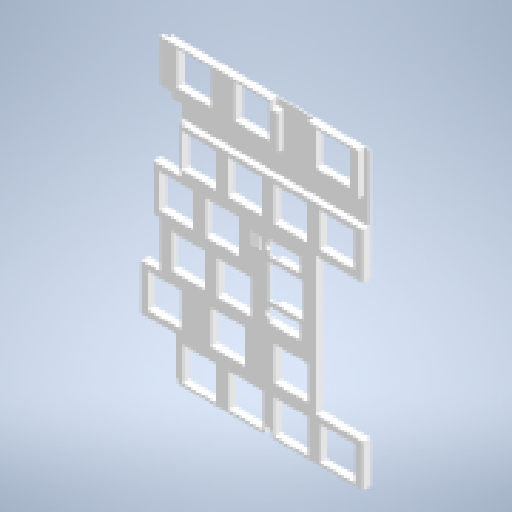
# Autodesk Inventor part: Right Plate
Saved by Autodesk Inventor 2025 (Build 290162000, 162)
## iProperties
Created: 2024-08-15
Part Number: Right Plate
Material: PBT Plastic
Document SubType Name: Modeling
Designer: adam
Density: 1.31 g/cm^3
Appearance: Smooth - White
Author: adam
Autodesk Inventor part; units mm, degrees
ref_plane "YZ Plane" through (0, 0, 0) normal (1, 0, 0) x (0, 1, 0)
ref_plane "XZ Plane" through (0, 0, 0) normal (0, 1, 0) x (-1, 0, 0)
ref_plane "XY Plane" through (0, 0, 0) normal (0, 0, 1) x (1, 0, 0)
sketch "Sketch1" plane through (0, 0, 0) normal (0, 0, 1) x (1, 0, 0)
  line L0 (356, -163) -> (40, -163) construction
  line L1 (356, -42) -> (356, -163) construction
  line L2 (40, -42) -> (356, -42) projected
  line L3 (40, -163) -> (40, -42) construction
  circle A0 centre (58.6, -159.6) radius 0.725 construction
  circle A1 centre (63, -154.9) radius 2.55 construction
  circle A2 centre (65.6, -160.65) radius 0.725 construction
  circle A3 centre (83.1, -159.6) radius 0.725 construction
  circle A4 centre (90.1, -160.65) radius 0.725 construction
  circle A5 centre (87.5, -154.9) radius 2.55 construction
  line L4 (107.125, -161.9) -> (113.125, -161.9) construction
  line L5 (107.125, -145.9) -> (107.125, -161.9) construction
  line L6 (113.125, -145.9) -> (107.125, -145.9) construction
  line L7 (113.125, -161.9) -> (113.125, -145.9) construction
  circle A6 centre (53.1, -140.5) radius 0.725 construction
  circle A7 centre (60.1, -141.55) radius 0.725 construction
  circle A8 centre (79.35, -140.5) radius 0.725 construction
  circle A9 centre (57.5, -135.8) radius 2.55 construction
  circle A10 centre (86.35, -141.55) radius 0.725 construction
  circle A11 centre (98.35, -140.5) radius 0.725 construction
  circle A12 centre (105.35, -141.55) radius 0.725 construction
  circle A13 centre (117.35, -140.5) radius 0.725 construction
  circle A14 centre (83.75, -135.8) radius 2.55 construction
  circle A15 centre (102.75, -135.8) radius 2.55 construction
  circle A16 centre (121.75, -135.8) radius 2.55 construction
  circle A17 centre (179.475, -160.65) radius 0.725 construction
  circle A18 centre (172.475, -159.6) radius 0.725 construction
  circle A19 centre (176.875, -154.9) radius 2.55 construction
  circle A20 centre (124.35, -141.55) radius 0.725 construction
  circle A21 centre (136.35, -140.5) radius 0.725 construction
  circle A22 centre (143.35, -141.55) radius 0.725 construction
  circle A23 centre (155.35, -140.5) radius 0.725 construction
  circle A24 centre (140.75, -135.8) radius 2.55 construction
  circle A25 centre (159.75, -135.8) radius 2.55 construction
  circle A26 centre (162.35, -141.55) radius 0.725 construction
  circle A27 centre (174.35, -140.5) radius 0.725 construction
  circle A28 centre (181.35, -141.55) radius 0.725 construction
  circle A29 centre (193.35, -140.5) radius 0.725 construction
  circle A30 centre (178.75, -135.8) radius 2.55 construction
  circle A31 centre (197.75, -135.8) radius 2.55 construction
  circle A32 centre (48.6, -121.4) radius 0.725 construction
  circle A33 centre (55.6, -122.45) radius 0.725 construction
  circle A34 centre (70.1, -121.4) radius 0.725 construction
  circle A35 centre (77.1, -122.45) radius 0.725 construction
  circle A36 centre (89.1, -121.4) radius 0.725 construction
  circle A37 centre (96.1, -122.45) radius 0.725 construction
  circle A38 centre (108.1, -121.4) radius 0.725 construction
  circle A39 centre (115.1, -122.45) radius 0.725 construction
  circle A40 centre (53, -116.7) radius 2.55 construction
  circle A41 centre (74.5, -116.7) radius 2.55 construction
  circle A42 centre (93.5, -116.7) radius 2.55 construction
  circle A43 centre (112.5, -116.7) radius 2.55 construction
  circle A44 centre (127.1, -121.4) radius 0.725 construction
  circle A45 centre (134.1, -122.45) radius 0.725 construction
  circle A46 centre (146.1, -121.4) radius 0.725 construction
  circle A47 centre (153.1, -122.45) radius 0.725 construction
  circle A48 centre (165.1, -121.4) radius 0.725 construction
  circle A49 centre (172.1, -122.45) radius 0.725 construction
  circle A50 centre (184.1, -121.4) radius 0.725 construction
  circle A51 centre (191.1, -122.45) radius 0.725 construction
  circle A52 centre (131.5, -116.7) radius 2.55 construction
  circle A53 centre (150.5, -116.7) radius 2.55 construction
  circle A54 centre (169.5, -116.7) radius 2.55 construction
  circle A55 centre (188.5, -116.7) radius 2.55 construction
  circle A56 centre (261.85, -159.6) radius 0.725 construction
  circle A57 centre (268.85, -160.65) radius 0.725 construction
  circle A58 centre (266.25, -154.9) radius 2.55 construction
  line L8 (240.625, -161.9) -> (246.625, -161.9) construction
  line L9 (240.625, -145.9) -> (240.625, -161.9) construction
  line L10 (246.625, -145.9) -> (240.625, -145.9) construction
  line L11 (246.625, -161.9) -> (246.625, -145.9) construction
  circle A59 centre (200.35, -141.55) radius 0.725 construction
  circle A60 centre (212.35, -140.5) radius 0.725 construction
  circle A61 centre (219.35, -141.55) radius 0.725 construction
  circle A62 centre (231.35, -140.5) radius 0.725 construction
  circle A63 centre (216.75, -135.8) radius 2.55 construction
  circle A64 centre (235.75, -135.8) radius 2.55 construction
  circle A65 centre (238.35, -141.55) radius 0.725 construction
  circle A66 centre (250.35, -140.5) radius 0.725 construction
  circle A67 centre (257.35, -141.55) radius 0.725 construction
  circle A68 centre (269.35, -140.5) radius 0.725 construction
  circle A69 centre (276.35, -141.55) radius 0.725 construction
  circle A70 centre (254.75, -135.8) radius 2.55 construction
  circle A71 centre (273.75, -135.8) radius 2.55 construction
  circle A72 centre (283.85, -159.6) radius 0.725 construction
  circle A73 centre (290.85, -160.65) radius 0.725 construction
  circle A74 centre (288.25, -154.9) radius 2.55 construction
  circle A75 centre (302.85, -159.6) radius 0.725 construction
  circle A76 centre (309.85, -160.65) radius 0.725 construction
  circle A77 centre (307.25, -154.9) radius 2.55 construction
  circle A78 centre (321.85, -159.6) radius 0.725 construction
  circle A79 centre (328.85, -160.65) radius 0.725 construction
  circle A80 centre (326.25, -154.9) radius 2.55 construction
  circle A81 centre (340.85, -159.6) radius 0.725 construction
  circle A82 centre (347.85, -160.65) radius 0.725 construction
  circle A83 centre (345.25, -154.9) radius 2.55 construction
  circle A84 centre (295.6, -140.5) radius 0.725 construction
  circle A85 centre (302.6, -141.55) radius 0.725 construction
  circle A86 centre (300, -135.8) radius 2.55 construction
  circle A87 centre (321.85, -140.5) radius 0.725 construction
  circle A88 centre (328.85, -141.55) radius 0.725 construction
  circle A89 centre (353.5, -141.62) radius 0.5 construction
  circle A90 centre (326.25, -135.8) radius 2.55 construction
  circle A91 centre (353.5, -139.08) radius 0.5 construction
  circle A92 centre (353.5, -136.54) radius 0.5 construction
  circle A93 centre (353.5, -134) radius 0.5 construction
  circle A94 centre (203.1, -121.4) radius 0.725 construction
  circle A95 centre (210.1, -122.45) radius 0.725 construction
  circle A96 centre (222.1, -121.4) radius 0.725 construction
  circle A97 centre (229.1, -122.45) radius 0.725 construction
  circle A98 centre (241.1, -121.4) radius 0.725 construction
  circle A99 centre (248.1, -122.45) radius 0.725 construction
  circle A100 centre (260.1, -121.4) radius 0.725 construction
  circle A101 centre (267.1, -122.45) radius 0.725 construction
  circle A102 centre (207.5, -116.7) radius 2.55 construction
  circle A103 centre (226.5, -116.7) radius 2.55 construction
  circle A104 centre (245.5, -116.7) radius 2.55 construction
  circle A105 centre (264.5, -116.7) radius 2.55 construction
  circle A106 centre (279.1, -121.4) radius 0.725 construction
  circle A107 centre (286.1, -122.45) radius 0.725 construction
  circle A108 centre (298.1, -121.4) radius 0.725 construction
  circle A109 centre (305.1, -122.45) radius 0.725 construction
  line L12 (315, -122.25) -> (330, -122.25) construction
  line L13 (315, -116.25) -> (315, -122.25) construction
  line L14 (330, -116.25) -> (315, -116.25) construction
  line L15 (330, -122.25) -> (330, -116.25) construction
  circle A110 centre (283.5, -116.7) radius 2.55 construction
  circle A111 centre (302.5, -116.7) radius 2.55 construction
  circle A112 centre (328.675, -111.675) radius 0.725 construction
  circle A113 centre (323.975, -107.275) radius 2.55 construction
  circle A114 centre (329.725, -104.675) radius 0.725 construction
  circle A115 centre (62.6, -103.35) radius 0.725 construction
  circle A116 centre (55.6, -102.3) radius 0.725 construction
  circle A117 centre (60, -97.6) radius 2.55 construction
  line L16 (45, -103.6) -> (51, -103.6) construction
  line L17 (45, -88.6) -> (45, -103.6) construction
  line L18 (51, -88.6) -> (45, -88.6) construction
  line L19 (51, -103.6) -> (51, -88.6) construction
  line L20 (69, -103.6) -> (75, -103.6) construction
  line L21 (69, -88.6) -> (69, -103.6) construction
  line L22 (75, -88.6) -> (69, -88.6) construction
  line L23 (75, -103.6) -> (75, -88.6) construction
  circle A118 centre (91.35, -103.35) radius 0.725 construction
  circle A119 centre (84.35, -102.3) radius 0.725 construction
  circle A120 centre (88.75, -97.6) radius 2.55 construction
  circle A121 centre (110.35, -103.35) radius 0.725 construction
  circle A122 centre (103.35, -102.3) radius 0.725 construction
  circle A123 centre (107.75, -97.6) radius 2.55 construction
  circle A124 centre (57.6, -84.25) radius 0.725 construction
  circle A125 centre (81.6, -84.25) radius 0.725 construction
  circle A126 centre (50.6, -83.2) radius 0.725 construction
  circle A127 centre (55, -78.5) radius 2.55 construction
  circle A128 centre (74.6, -83.2) radius 0.725 construction
  circle A129 centre (79, -78.5) radius 2.55 construction
  circle A130 centre (100.6, -84.25) radius 0.725 construction
  circle A131 centre (119.6, -84.25) radius 0.725 construction
  circle A132 centre (93.6, -83.2) radius 0.725 construction
  circle A133 centre (98, -78.5) radius 2.55 construction
  circle A134 centre (112.6, -83.2) radius 0.725 construction
  circle A135 centre (117, -78.5) radius 2.55 construction
  circle A136 centre (129.35, -103.35) radius 0.725 construction
  circle A137 centre (122.35, -102.3) radius 0.725 construction
  circle A138 centre (141.35, -102.3) radius 0.725 construction
  circle A139 centre (126.75, -97.6) radius 2.55 construction
  circle A140 centre (148.35, -103.35) radius 0.725 construction
  circle A141 centre (160.35, -102.3) radius 0.725 construction
  circle A142 centre (145.75, -97.6) radius 2.55 construction
  circle A143 centre (167.35, -103.35) radius 0.725 construction
  circle A144 centre (179.35, -102.3) radius 0.725 construction
  circle A145 centre (164.75, -97.6) radius 2.55 construction
  circle A146 centre (186.35, -103.35) radius 0.725 construction
  circle A147 centre (198.35, -102.3) radius 0.725 construction
  circle A148 centre (183.75, -97.6) radius 2.55 construction
  circle A149 centre (138.6, -84.25) radius 0.725 construction
  circle A150 centre (157.6, -84.25) radius 0.725 construction
  circle A151 centre (131.6, -83.2) radius 0.725 construction
  circle A152 centre (136, -78.5) radius 2.55 construction
  circle A153 centre (150.6, -83.2) radius 0.725 construction
  circle A154 centre (155, -78.5) radius 2.55 construction
  circle A155 centre (176.6, -84.25) radius 0.725 construction
  circle A156 centre (195.6, -84.25) radius 0.725 construction
  circle A157 centre (169.6, -83.2) radius 0.725 construction
  circle A158 centre (174, -78.5) radius 2.55 construction
  circle A159 centre (188.6, -83.2) radius 0.725 construction
  circle A160 centre (193, -78.5) radius 2.55 construction
  circle A161 centre (48.1, -54.7) radius 0.725 construction
  circle A162 centre (55.1, -55.75) radius 0.725 construction
  circle A163 centre (81.1, -54.7) radius 0.725 construction
  circle A164 centre (52.5, -50) radius 2.55 construction
  circle A165 centre (88.1, -55.75) radius 0.725 construction
  circle A166 centre (105.1, -54.7) radius 0.725 construction
  circle A167 centre (112.1, -55.75) radius 0.725 construction
  circle A168 centre (85.5, -50) radius 2.55 construction
  circle A169 centre (109.5, -50) radius 2.55 construction
  circle A170 centre (163.5, -66.25) radius 0.425 construction
  circle A171 centre (166, -66.25) radius 0.425 construction
  circle A172 centre (168.5, -66.25) radius 0.425 construction
  circle A173 centre (171, -66.25) radius 0.425 construction
  circle A174 centre (173.5, -66.25) radius 0.425 construction
  circle A175 centre (176, -66.25) radius 0.425 construction
  circle A176 centre (178.5, -66.25) radius 0.425 construction
  circle A177 centre (162.25, -63.75) radius 0.425 construction
  circle A178 centre (164.75, -63.75) radius 0.425 construction
  circle A179 centre (167.25, -63.75) radius 0.425 construction
  circle A180 centre (169.75, -63.75) radius 0.425 construction
  circle A181 centre (172.25, -63.75) radius 0.425 construction
  circle A182 centre (174.75, -63.75) radius 0.425 construction
  circle A183 centre (177.25, -63.75) radius 0.425 construction
  circle A184 centre (179.75, -63.75) radius 0.425 construction
  circle A185 centre (181, -66.25) radius 0.425 construction
  circle A186 centre (183.5, -66.25) radius 0.425 construction
  circle A187 centre (186, -66.25) radius 0.425 construction
  circle A188 centre (188.5, -66.25) radius 0.425 construction
  circle A189 centre (191, -66.25) radius 0.425 construction
  circle A190 centre (193.5, -66.25) radius 0.425 construction
  circle A191 centre (196, -66.25) radius 0.425 construction
  circle A192 centre (198.5, -66.25) radius 0.425 construction
  circle A193 centre (182.25, -63.75) radius 0.425 construction
  circle A194 centre (184.75, -63.75) radius 0.425 construction
  circle A195 centre (187.25, -63.75) radius 0.425 construction
  circle A196 centre (189.75, -63.75) radius 0.425 construction
  circle A197 centre (192.25, -63.75) radius 0.425 construction
  circle A198 centre (194.75, -63.75) radius 0.425 construction
  circle A199 centre (197.25, -63.75) radius 0.425 construction
  circle A200 centre (129.1, -54.7) radius 0.725 construction
  circle A201 centre (136.1, -55.75) radius 0.725 construction
  circle A202 centre (153.1, -54.7) radius 0.725 construction
  circle A203 centre (160.1, -55.75) radius 0.725 construction
  circle A204 centre (133.5, -50) radius 2.55 construction
  circle A205 centre (157.5, -50) radius 2.55 construction
  circle A206 centre (177.1, -54.7) radius 0.725 construction
  circle A207 centre (184.1, -55.75) radius 0.725 construction
  circle A208 centre (181.5, -50) radius 2.55 construction
  circle A209 centre (205.35, -103.35) radius 0.725 construction
  circle A210 centre (217.35, -102.3) radius 0.725 construction
  circle A211 centre (202.75, -97.6) radius 2.55 construction
  circle A212 centre (224.35, -103.35) radius 0.725 construction
  circle A213 centre (236.35, -102.3) radius 0.725 construction
  circle A214 centre (221.75, -97.6) radius 2.55 construction
  circle A215 centre (243.35, -103.35) radius 0.725 construction
  circle A216 centre (255.35, -102.3) radius 0.725 construction
  circle A217 centre (240.75, -97.6) radius 2.55 construction
  circle A218 centre (262.35, -103.35) radius 0.725 construction
  circle A219 centre (274.35, -102.3) radius 0.725 construction
  circle A220 centre (259.75, -97.6) radius 2.55 construction
  circle A221 centre (214.6, -84.25) radius 0.725 construction
  circle A222 centre (233.6, -84.25) radius 0.725 construction
  circle A223 centre (207.6, -83.2) radius 0.725 construction
  circle A224 centre (212, -78.5) radius 2.55 construction
  circle A225 centre (226.6, -83.2) radius 0.725 construction
  circle A226 centre (231, -78.5) radius 2.55 construction
  circle A227 centre (252.6, -84.25) radius 0.725 construction
  circle A228 centre (271.6, -84.25) radius 0.725 construction
  circle A229 centre (245.6, -83.2) radius 0.725 construction
  circle A230 centre (250, -78.5) radius 2.55 construction
  circle A231 centre (264.6, -83.2) radius 0.725 construction
  circle A232 centre (269, -78.5) radius 2.55 construction
  circle A233 centre (281.35, -103.35) radius 0.725 construction
  circle A234 centre (293.35, -102.3) radius 0.725 construction
  circle A235 centre (278.75, -97.6) radius 2.55 construction
  circle A236 centre (300.35, -103.35) radius 0.725 construction
  circle A237 centre (297.75, -97.6) radius 2.55 construction
  line L24 (315, -98.25) -> (330, -98.25) construction
  line L25 (315, -92.25) -> (315, -98.25) construction
  line L26 (330, -92.25) -> (315, -92.25) construction
  line L27 (330, -98.25) -> (330, -92.25) construction
  circle A238 centre (290.6, -84.25) radius 0.725 construction
  circle A239 centre (309.6, -84.25) radius 0.725 construction
  circle A240 centre (283.6, -83.2) radius 0.725 construction
  circle A241 centre (288, -78.5) radius 2.55 construction
  circle A242 centre (302.6, -83.2) radius 0.725 construction
  circle A243 centre (307, -78.5) radius 2.55 construction
  circle A244 centre (328.6, -84.25) radius 0.725 construction
  circle A245 centre (347.6, -84.25) radius 0.725 construction
  circle A246 centre (321.6, -83.2) radius 0.725 construction
  circle A247 centre (326, -78.5) radius 2.55 construction
  circle A248 centre (340.6, -83.2) radius 0.725 construction
  circle A249 centre (345, -78.5) radius 2.55 construction
  circle A250 centre (201, -66.25) radius 0.425 construction
  circle A251 centre (199.75, -63.75) radius 0.425 construction
  circle A252 centre (259, -74) radius 1.6 construction
  circle A253 centre (209.6, -54.7) radius 0.725 construction
  circle A254 centre (216.6, -55.75) radius 0.725 construction
  circle A255 centre (233.6, -54.7) radius 0.725 construction
  circle A256 centre (214, -50) radius 2.55 construction
  circle A257 centre (238, -50) radius 2.55 construction
  circle A258 centre (240.6, -55.75) radius 0.725 construction
  circle A259 centre (257.6, -54.7) radius 0.725 construction
  circle A260 centre (264.6, -55.75) radius 0.725 construction
  circle A261 centre (262, -50) radius 2.55 construction
  circle A262 centre (281.6, -54.7) radius 0.725 construction
  circle A263 centre (288.6, -55.75) radius 0.725 construction
  circle A264 centre (305.6, -54.7) radius 0.725 construction
  circle A265 centre (312.6, -55.75) radius 0.725 construction
  circle A266 centre (286, -50) radius 2.55 construction
  circle A267 centre (310, -50) radius 2.55 construction
  circle A268 centre (339.1, -54.7) radius 0.725 construction
  circle A269 centre (346.1, -55.75) radius 0.725 construction
  circle A270 centre (343.5, -50) radius 2.55 construction
  line L28 (274, -42) -> (274, -64.25) projected
  line L29 (274, -64.25) -> (278.5, -64.25) projected
  line L30 (278.5, -88.05) -> (278.5, -64.25) projected
  line L31 (269.25, -88.05) -> (278.5, -88.05) projected
  line L32 (269.25, -107.15) -> (269.25, -88.05) projected
  line L33 (274, -107.15) -> (269.25, -107.15) projected
  line L34 (274, -126.25) -> (274, -107.15) projected
  line L35 (264.25, -126.25) -> (274, -126.25) projected
  line L36 (264.25, -145.35) -> (264.25, -126.25) projected
  line L37 (277.25, -145.35) -> (264.25, -145.35) projected
  line L38 (277.25, -163) -> (277.25, -145.35) projected
  line L39 (274, -42) -> (356, -42) construction
  line L40 (356, -42) -> (356, -163)
  line L41 (356, -163) -> (277.25, -163)
  line L42 (278.9975, -42.9975) -> (293.0025, -42.9975)
  line L43 (293.0025, -42.9975) -> (293.0025, -57.0025)
  line L44 (293.0025, -57.0025) -> (278.9975, -57.0025)
  line L45 (278.9975, -57.0025) -> (278.9975, -42.9975)
  line L46 (278.9975, -42.9975) -> (293.0025, -57.0025) construction
  line L47 (293.0025, -42.9975) -> (278.9975, -57.0025) construction
  line L48 (302.9975, -42.9975) -> (317.0025, -42.9975)
  line L49 (317.0025, -42.9975) -> (317.0025, -57.0025)
  line L50 (317.0025, -57.0025) -> (302.9975, -57.0025)
  line L51 (302.9975, -57.0025) -> (302.9975, -42.9975)
  line L52 (302.9975, -42.9975) -> (317.0025, -57.0025) construction
  line L53 (317.0025, -42.9975) -> (302.9975, -57.0025) construction
  line L54 (336.4975, -42.9975) -> (350.5025, -42.9975)
  line L55 (350.5025, -42.9975) -> (350.5025, -57.0025)
  line L56 (350.5025, -57.0025) -> (336.4975, -57.0025)
  line L57 (336.4975, -57.0025) -> (336.4975, -42.9975)
  line L58 (336.4975, -42.9975) -> (350.5025, -57.0025) construction
  line L59 (350.5025, -42.9975) -> (336.4975, -57.0025) construction
  line L60 (280.9975, -71.4975) -> (295.0025, -71.4975)
  line L61 (295.0025, -71.4975) -> (295.0025, -85.5025)
  line L62 (295.0025, -85.5025) -> (280.9975, -85.5025)
  line L63 (280.9975, -85.5025) -> (280.9975, -71.4975)
  line L64 (280.9975, -71.4975) -> (295.0025, -85.5025) construction
  line L65 (295.0025, -71.4975) -> (280.9975, -85.5025) construction
  line L66 (299.9975, -71.4975) -> (314.0025, -71.4975)
  line L67 (314.0025, -71.4975) -> (314.0025, -85.5025)
  line L68 (314.0025, -85.5025) -> (299.9975, -85.5025)
  line L69 (299.9975, -85.5025) -> (299.9975, -71.4975)
  line L70 (299.9975, -71.4975) -> (314.0025, -85.5025) construction
  line L71 (314.0025, -71.4975) -> (299.9975, -85.5025) construction
  line L72 (318.9975, -71.4975) -> (333.0025, -71.4975)
  line L73 (333.0025, -71.4975) -> (333.0025, -85.5025)
  line L74 (333.0025, -85.5025) -> (318.9975, -85.5025)
  line L75 (318.9975, -85.5025) -> (318.9975, -71.4975)
  line L76 (318.9975, -71.4975) -> (333.0025, -85.5025) construction
  line L77 (333.0025, -71.4975) -> (318.9975, -85.5025) construction
  line L78 (337.9975, -71.4975) -> (352.0025, -71.4975)
  line L79 (352.0025, -71.4975) -> (352.0025, -85.5025)
  line L80 (352.0025, -85.5025) -> (337.9975, -85.5025)
  line L81 (337.9975, -85.5025) -> (337.9975, -71.4975)
  line L82 (337.9975, -71.4975) -> (352.0025, -85.5025) construction
  line L83 (352.0025, -71.4975) -> (337.9975, -85.5025) construction
  line L84 (271.7475, -90.5975) -> (285.7525, -90.5975)
  line L85 (285.7525, -90.5975) -> (285.7525, -104.6025)
  line L86 (285.7525, -104.6025) -> (271.7475, -104.6025)
  line L87 (271.7475, -104.6025) -> (271.7475, -90.5975)
  line L88 (271.7475, -90.5975) -> (285.7525, -104.6025) construction
  line L89 (285.7525, -90.5975) -> (271.7475, -104.6025) construction
  line L90 (290.7475, -90.5975) -> (304.7525, -90.5975)
  line L91 (304.7525, -90.5975) -> (304.7525, -104.6025)
  line L92 (304.7525, -104.6025) -> (290.7475, -104.6025)
  line L93 (290.7475, -104.6025) -> (290.7475, -90.5975)
  line L94 (290.7475, -90.5975) -> (304.7525, -104.6025) construction
  line L95 (304.7525, -90.5975) -> (290.7475, -104.6025) construction
  line L96 (316.9725, -100.2725) -> (330.9775, -100.2725)
  line L97 (330.9775, -100.2725) -> (330.9775, -114.2775)
  line L98 (330.9775, -114.2775) -> (316.9725, -114.2775)
  line L99 (316.9725, -114.2775) -> (316.9725, -100.2725)
  line L100 (316.9725, -100.2725) -> (330.9775, -114.2775) construction
  line L101 (330.9775, -100.2725) -> (316.9725, -114.2775) construction
  line L102 (295.4975, -109.6975) -> (309.5025, -109.6975)
  line L103 (309.5025, -109.6975) -> (309.5025, -123.7025)
  line L104 (309.5025, -123.7025) -> (295.4975, -123.7025)
  line L105 (295.4975, -123.7025) -> (295.4975, -109.6975)
  line L106 (295.4975, -109.6975) -> (309.5025, -123.7025) construction
  line L107 (309.5025, -109.6975) -> (295.4975, -123.7025) construction
  line L108 (276.4975, -109.6975) -> (290.5025, -109.6975)
  line L109 (290.5025, -109.6975) -> (290.5025, -123.7025)
  line L110 (290.5025, -123.7025) -> (276.4975, -123.7025)
  line L111 (276.4975, -123.7025) -> (276.4975, -109.6975)
  line L112 (276.4975, -109.6975) -> (290.5025, -123.7025) construction
  line L113 (290.5025, -109.6975) -> (276.4975, -123.7025) construction
  line L114 (266.7475, -128.7975) -> (280.7525, -128.7975)
  line L115 (280.7525, -128.7975) -> (280.7525, -142.8025)
  line L116 (280.7525, -142.8025) -> (266.7475, -142.8025)
  line L117 (266.7475, -142.8025) -> (266.7475, -128.7975)
  line L118 (266.7475, -128.7975) -> (280.7525, -142.8025) construction
  line L119 (280.7525, -128.7975) -> (266.7475, -142.8025) construction
  line L120 (292.9975, -128.7975) -> (307.0025, -128.7975)
  line L121 (307.0025, -128.7975) -> (307.0025, -142.8025)
  line L122 (307.0025, -142.8025) -> (292.9975, -142.8025)
  line L123 (292.9975, -142.8025) -> (292.9975, -128.7975)
  line L124 (292.9975, -128.7975) -> (307.0025, -142.8025) construction
  line L125 (307.0025, -128.7975) -> (292.9975, -142.8025) construction
  line L126 (319.2475, -128.7975) -> (333.2525, -128.7975)
  line L127 (333.2525, -128.7975) -> (333.2525, -142.8025)
  line L128 (333.2525, -142.8025) -> (319.2475, -142.8025)
  line L129 (319.2475, -142.8025) -> (319.2475, -128.7975)
  line L130 (319.2475, -128.7975) -> (333.2525, -142.8025) construction
  line L131 (333.2525, -128.7975) -> (319.2475, -142.8025) construction
  line L132 (281.2475, -147.8975) -> (295.2525, -147.8975)
  line L133 (295.2525, -147.8975) -> (295.2525, -161.9025)
  line L134 (295.2525, -161.9025) -> (281.2475, -161.9025)
  line L135 (281.2475, -161.9025) -> (281.2475, -147.8975)
  line L136 (281.2475, -147.8975) -> (295.2525, -161.9025) construction
  line L137 (295.2525, -147.8975) -> (281.2475, -161.9025) construction
  line L138 (300.2475, -147.8975) -> (314.2525, -147.8975)
  line L139 (314.2525, -147.8975) -> (314.2525, -161.9025)
  line L140 (314.2525, -161.9025) -> (300.2475, -161.9025)
  line L141 (300.2475, -161.9025) -> (300.2475, -147.8975)
  line L142 (300.2475, -147.8975) -> (314.2525, -161.9025) construction
  line L143 (314.2525, -147.8975) -> (300.2475, -161.9025) construction
  line L144 (319.2475, -147.8975) -> (333.2525, -147.8975)
  line L145 (333.2525, -147.8975) -> (333.2525, -161.9025)
  line L146 (333.2525, -161.9025) -> (319.2475, -161.9025)
  line L147 (319.2475, -161.9025) -> (319.2475, -147.8975)
  line L148 (319.2475, -147.8975) -> (333.2525, -161.9025) construction
  line L149 (333.2525, -147.8975) -> (319.2475, -161.9025) construction
  line L150 (338.2475, -147.8975) -> (352.2525, -147.8975)
  line L151 (352.2525, -147.8975) -> (352.2525, -161.9025)
  line L152 (352.2525, -161.9025) -> (338.2475, -161.9025)
  line L153 (338.2475, -161.9025) -> (338.2475, -147.8975)
  line L154 (338.2475, -147.8975) -> (352.2525, -161.9025) construction
  line L155 (352.2525, -147.8975) -> (338.2475, -161.9025) construction
  line L156 (317.2225, -92.25) -> (317.2225, -94.25)
  line L157 (317.2225, -94.25) -> (315.7225, -94.25)
  line L158 (315.7225, -94.25) -> (315.7225, -96.25)
  line L159 (315.7225, -96.25) -> (317.2225, -96.25)
  line L160 (317.2225, -96.25) -> (317.2225, -98.25)
  line L161 (317.2225, -98.25) -> (329.7225, -98.25)
  line L162 (329.7225, -98.25) -> (329.7225, -92.25)
  line L163 (329.7225, -92.25) -> (317.2225, -92.25)
  line L164 (315.0875, -122.25) -> (330.0875, -122.25) construction
  line L165 (315.0875, -116.25) -> (315.0875, -122.25) construction
  line L166 (330.0875, -116.25) -> (315.0875, -116.25) construction
  line L167 (317.2225, -116.25) -> (317.2225, -118.25)
  line L168 (317.2225, -118.25) -> (315.7225, -118.25)
  line L169 (315.7225, -118.25) -> (315.7225, -120.25)
  line L170 (315.7225, -120.25) -> (317.2225, -120.25)
  line L171 (317.2225, -120.25) -> (317.2225, -122.25)
  line L172 (317.2225, -122.25) -> (329.7225, -122.25)
  line L173 (329.7225, -122.25) -> (329.7225, -116.25)
  line L174 (329.7225, -116.25) -> (317.2225, -116.25)
  line L175 (356, -145.5) -> (336.5, -145.5)
  line L176 (336.5, -145.5) -> (336.5, -88.5)
  line L177 (336.5, -88.5) -> (356, -88.5)
  line L178 (356, -88.5) -> (356, -145.5)
  point P0 (0, 0)
  dimension "d0" = 14.005
  dimension "d1" = 14.005
  dimension "d2" = 14.005
  dimension "d3" = 14.005
  dimension "d4" = 14.005
  dimension "d5" = 14.005
  dimension "d6" = 14.005
  dimension "d7" = 14.005
  dimension "d8" = 14.005
  dimension "d9" = 14.005
  dimension "d10" = 14.005
  dimension "d11" = 14.005
  dimension "d12" = 14.005
  dimension "d13" = 14.005
  dimension "d14" = 14.005
  dimension "d15" = 14.005
  dimension "d16" = 14.005
  dimension "d17" = 14.005
  dimension "d18" = 14.005
  dimension "d19" = 14.005
  dimension "d20" = 14.005
  dimension "d21" = 14.005
  dimension "d22" = 14.005
  dimension "d23" = 14.005
  dimension "d24" = 14.005
  dimension "d25" = 14.005
  dimension "d26" = 14.005
  dimension "d27" = 14.005
  dimension "d28" = 14.005
  dimension "d29" = 14.005
  dimension "d30" = 14.005
  dimension "d31" = 14.005
  dimension "d32" = 14.005
  dimension "d33" = 14.005
  dimension "d34" = 14.005
  dimension "d35" = 14.005
  dimension "d36" = 14.005
  dimension "d37" = 14.005
  dimension "d38" = 12.5
  dimension "d39" = 2
  dimension "d40" = 1.5
  dimension "d42" = 12.5
  dimension "d43" = 2
  dimension "d44" = 1.5
  dimension "d65" = 17.5
  dimension "d66" = 74.5
  dimension "d67" = 19.5
  dimension "d81" = 0.25
  constraints: 280 end point, 38 midpoint, 38 parallel, 30 perpendicular, 19 horizontal, 14 point on line, 10 collinear, 3 vertical
  measures "d0" distance of L43.end L44.end
  measures "d1" distance of L42.end L43.end
  measures "d2" distance of L49.end L50.end
  measures "d3" distance of L48.end L49.end
  measures "d4" distance of L55.end L56.end
  measures "d5" distance of L54.end L55.end
  measures "d6" distance of L61.end L62.end
  measures "d7" distance of L60.end L61.end
  measures "d8" distance of L67.end L68.end
  measures "d9" distance of L66.end L67.end
  measures "d10" distance of L73.end L74.end
  measures "d11" distance of L72.end L73.end
  measures "d12" distance of L79.end L80.end
  measures "d13" distance of L78.end L79.end
  measures "d14" distance of L85.end L86.end
  measures "d15" distance of L84.end L85.end
  measures "d16" distance of L91.end L92.end
  measures "d17" distance of L90.end L91.end
  measures "d18" distance of L97.end L98.end
  measures "d19" distance of L96.end L97.end
  measures "d20" distance of L103.end L104.end
  measures "d21" distance of L102.end L103.end
  measures "d22" distance of L109.end L110.end
  measures "d23" distance of L108.end L109.end
  measures "d24" distance of L115.end L116.end
  measures "d25" distance of L114.end L115.end
  measures "d26" distance of L121.end L122.end
  measures "d27" distance of L120.end L121.end
  measures "d28" distance of L127.end L128.end
  measures "d29" distance of L126.end L127.end
  measures "d30" distance of L133.end L134.end
  measures "d31" distance of L132.end L133.end
  measures "d32" distance of L139.end L140.end
  measures "d33" distance of L138.end L139.end
  measures "d34" distance of L145.end L146.end
  measures "d35" distance of L144.end L145.end
  measures "d36" distance of L151.end L152.end
  measures "d37" distance of L150.end L151.end
  measures "d38" distance between parallel lines of L162 L156
  measures "d39" distance of L157.end L158.end
  measures "d40" distance of L156.end L157.end
  measures "d42" distance between parallel lines of L173 L167
  measures "d43" distance of L168.end L169.end
  measures "d44" distance of L167.end L168.end
  measures "d65" distance between parallel lines of L175 L0
  measures "d66" distance between parallel lines of L177 L41
  measures "d67" distance between parallel lines of L1 L176
  measures "d81" distance between parallel lines of L160 L99
extrude "Extrusion1" add sketch "Sketch1" along normal blind 0.5 contours L2 L40 L177 L176 L175 L41 L38 L37 L36 L35 L34 L33 L32 L31 L30 L29 L28
sketch "Sketch2" plane through (0, 0, 0.5) normal (0, 0, 1) x (1, 0, 0)
  line L0 (356, -42) -> (274, -42) projected
  line L1 (332.9975, -42) -> (332.9975, -59.5)
  line L2 (332.9975, -59.5) -> (354.0025, -59.5)
  line L3 (354.0025, -59.5) -> (354.0025, -42)
  line L4 (320.5025, -42) -> (320.5025, -59.5)
  line L5 (320.5025, -59.5) -> (274, -59.5)
  line L6 (278.5, -64.25) -> (278.5, -88.05) projected
  line L7 (278.5, -69.5) -> (356, -69.5)
  line L8 (356, -163) -> (356, -42) projected
  line L9 (356, -88.5) -> (336.5, -88.5)
  line L10 (336.5, -88.5) -> (336.5, -145.5)
  line L11 (336.5, -145.5) -> (356, -145.5)
  line L12 (277.25, -163) -> (356, -163) projected
  line L13 (350.5025, -42.9975) -> (350.5025, -57.0025) projected
  line L14 (336.4975, -57.0025) -> (336.4975, -42.9975) projected
  line L15 (317.0025, -42.9975) -> (317.0025, -57.0025) projected
  line L16 (278.5, -64.25) -> (278.5, -88.05) projected
  line L17 (278.5, -88.05) -> (269.25, -88.05) projected
  line L18 (269.25, -88.05) -> (269.25, -107.15) projected
  line L19 (269.25, -107.15) -> (274, -107.15) projected
  line L20 (274, -107.15) -> (274, -126.25) projected
  line L21 (274, -126.25) -> (264.25, -126.25) projected
  line L22 (264.25, -126.25) -> (264.25, -145.35) projected
  line L23 (264.25, -145.35) -> (277.25, -145.35) projected
  line L24 (277.25, -145.35) -> (277.25, -163) projected
  line L25 (277.25, -163) -> (356, -163) projected
  line L26 (356, -163) -> (356, -145.5) projected
  line L27 (356, -42) -> (274, -42) projected
  line L28 (274, -42) -> (274, -64.25) projected
  line L29 (274, -64.25) -> (278.5, -64.25) projected
  line L30 (329.7225, -122.25) -> (317.2225, -122.25) projected
  line L31 (317.2225, -122.25) -> (317.2225, -120.25) projected
  line L32 (317.2225, -120.25) -> (315.7225, -120.25) projected
  line L33 (315.7225, -120.25) -> (315.7225, -118.25) projected
  line L34 (315.7225, -118.25) -> (317.2225, -118.25) projected
  line L35 (317.2225, -118.25) -> (317.2225, -116.25) projected
  line L36 (317.2225, -116.25) -> (329.7225, -116.25) projected
  line L37 (329.7225, -116.25) -> (329.7225, -122.25) projected
  line L38 (317.2225, -92.25) -> (329.7225, -92.25) projected
  line L39 (329.7225, -92.25) -> (329.7225, -98.25) projected
  line L40 (329.7225, -98.25) -> (317.2225, -98.25) projected
  line L41 (317.2225, -98.25) -> (317.2225, -96.25) projected
  line L42 (317.2225, -96.25) -> (315.7225, -96.25) projected
  line L43 (315.7225, -96.25) -> (315.7225, -94.25) projected
  line L44 (315.7225, -94.25) -> (317.2225, -94.25) projected
  line L45 (317.2225, -94.25) -> (317.2225, -92.25) projected
  line L46 (338.2475, -147.8975) -> (352.2525, -147.8975) projected
  line L47 (352.2525, -147.8975) -> (352.2525, -161.9025) projected
  line L48 (352.2525, -161.9025) -> (338.2475, -161.9025) projected
  line L49 (338.2475, -161.9025) -> (338.2475, -147.8975) projected
  line L50 (319.2475, -147.8975) -> (333.2525, -147.8975) projected
  line L51 (333.2525, -147.8975) -> (333.2525, -161.9025) projected
  line L52 (333.2525, -161.9025) -> (319.2475, -161.9025) projected
  line L53 (319.2475, -161.9025) -> (319.2475, -147.8975) projected
  line L54 (300.2475, -147.8975) -> (314.2525, -147.8975) projected
  line L55 (314.2525, -147.8975) -> (314.2525, -161.9025) projected
  line L56 (314.2525, -161.9025) -> (300.2475, -161.9025) projected
  line L57 (300.2475, -161.9025) -> (300.2475, -147.8975) projected
  line L58 (281.2475, -147.8975) -> (295.2525, -147.8975) projected
  line L59 (295.2525, -147.8975) -> (295.2525, -161.9025) projected
  line L60 (295.2525, -161.9025) -> (281.2475, -161.9025) projected
  line L61 (281.2475, -161.9025) -> (281.2475, -147.8975) projected
  line L62 (319.2475, -128.7975) -> (333.2525, -128.7975) projected
  line L63 (333.2525, -128.7975) -> (333.2525, -142.8025) projected
  line L64 (333.2525, -142.8025) -> (319.2475, -142.8025) projected
  line L65 (319.2475, -142.8025) -> (319.2475, -128.7975) projected
  line L66 (292.9975, -128.7975) -> (307.0025, -128.7975) projected
  line L67 (307.0025, -128.7975) -> (307.0025, -142.8025) projected
  line L68 (307.0025, -142.8025) -> (292.9975, -142.8025) projected
  line L69 (292.9975, -142.8025) -> (292.9975, -128.7975) projected
  line L70 (266.7475, -128.7975) -> (280.7525, -128.7975) projected
  line L71 (280.7525, -128.7975) -> (280.7525, -142.8025) projected
  line L72 (280.7525, -142.8025) -> (266.7475, -142.8025) projected
  line L73 (266.7475, -142.8025) -> (266.7475, -128.7975) projected
  line L74 (276.4975, -109.6975) -> (290.5025, -109.6975) projected
  line L75 (290.5025, -109.6975) -> (290.5025, -123.7025) projected
  line L76 (290.5025, -123.7025) -> (276.4975, -123.7025) projected
  line L77 (276.4975, -123.7025) -> (276.4975, -109.6975) projected
  line L78 (295.4975, -109.6975) -> (309.5025, -109.6975) projected
  line L79 (309.5025, -109.6975) -> (309.5025, -123.7025) projected
  line L80 (309.5025, -123.7025) -> (295.4975, -123.7025) projected
  line L81 (295.4975, -123.7025) -> (295.4975, -109.6975) projected
  line L82 (316.9725, -100.2725) -> (330.9775, -100.2725) projected
  line L83 (330.9775, -100.2725) -> (330.9775, -114.2775) projected
  line L84 (330.9775, -114.2775) -> (316.9725, -114.2775) projected
  line L85 (316.9725, -114.2775) -> (316.9725, -100.2725) projected
  line L86 (290.7475, -90.5975) -> (304.7525, -90.5975) projected
  line L87 (304.7525, -90.5975) -> (304.7525, -104.6025) projected
  line L88 (304.7525, -104.6025) -> (290.7475, -104.6025) projected
  line L89 (290.7475, -104.6025) -> (290.7475, -90.5975) projected
  line L90 (271.7475, -90.5975) -> (285.7525, -90.5975) projected
  line L91 (285.7525, -90.5975) -> (285.7525, -104.6025) projected
  line L92 (285.7525, -104.6025) -> (271.7475, -104.6025) projected
  line L93 (271.7475, -104.6025) -> (271.7475, -90.5975) projected
  line L94 (337.9975, -71.4975) -> (352.0025, -71.4975) projected
  line L95 (352.0025, -71.4975) -> (352.0025, -85.5025) projected
  line L96 (352.0025, -85.5025) -> (337.9975, -85.5025) projected
  line L97 (337.9975, -85.5025) -> (337.9975, -71.4975) projected
  line L98 (318.9975, -71.4975) -> (333.0025, -71.4975) projected
  line L99 (333.0025, -71.4975) -> (333.0025, -85.5025) projected
  line L100 (333.0025, -85.5025) -> (318.9975, -85.5025) projected
  line L101 (318.9975, -85.5025) -> (318.9975, -71.4975) projected
  line L102 (299.9975, -71.4975) -> (314.0025, -71.4975) projected
  line L103 (314.0025, -71.4975) -> (314.0025, -85.5025) projected
  line L104 (314.0025, -85.5025) -> (299.9975, -85.5025) projected
  line L105 (299.9975, -85.5025) -> (299.9975, -71.4975) projected
  line L106 (280.9975, -71.4975) -> (295.0025, -71.4975) projected
  line L107 (295.0025, -71.4975) -> (295.0025, -85.5025) projected
  line L108 (295.0025, -85.5025) -> (280.9975, -85.5025) projected
  line L109 (280.9975, -85.5025) -> (280.9975, -71.4975) projected
  line L110 (336.4975, -42.9975) -> (350.5025, -42.9975) projected
  line L111 (350.5025, -42.9975) -> (350.5025, -57.0025) projected
  line L112 (350.5025, -57.0025) -> (336.4975, -57.0025) projected
  line L113 (336.4975, -57.0025) -> (336.4975, -42.9975) projected
  line L114 (302.9975, -42.9975) -> (317.0025, -42.9975) projected
  line L115 (317.0025, -42.9975) -> (317.0025, -57.0025) projected
  line L116 (317.0025, -57.0025) -> (302.9975, -57.0025) projected
  line L117 (302.9975, -57.0025) -> (302.9975, -42.9975) projected
  line L118 (278.9975, -42.9975) -> (293.0025, -42.9975) projected
  line L119 (293.0025, -42.9975) -> (293.0025, -57.0025) projected
  line L120 (293.0025, -57.0025) -> (278.9975, -57.0025) projected
  line L121 (278.9975, -57.0025) -> (278.9975, -42.9975) projected
  line L122 (356, -145.5) -> (336.5, -145.5) projected
  line L123 (336.5, -145.5) -> (336.5, -88.5) projected
  line L124 (336.5, -88.5) -> (356, -88.5) projected
  line L125 (356, -88.5) -> (356, -42) projected
  point P0 (0, 0)
  dimension "d47" = 17.5
  dimension "d48" = 74.5
  dimension "d49" = 93.5
  dimension "d50" = 103.5
  dimension "d51" = 3.5
  dimension "d52" = 3.5
  dimension "d53" = 3.5
  dimension "d54" = 19.5
  constraints: 18 end point, 8 point on line, 4 perpendicular, 2 horizontal, 1 parallel, 1 vertical
  measures "d47" distance between parallel lines of L12 L11
  measures "d48" distance between parallel lines of L12 L9
  measures "d49" distance between parallel lines of L7 L12
  measures "d50" distance between parallel lines of L12 L2
  measures "d51" distance between parallel lines of L3 L13
  measures "d52" distance between parallel lines of L14 L1
  measures "d53" distance between parallel lines of L4 L15
  measures "d54" distance between parallel lines of L8 L10
extrude "Extrusion2" add sketch "Sketch2" along normal blind 2.5 contours L3 L2 L1 L0 | L8 L9 L10 L11 L12 L24 L23 L22 L21 L20 L19 L18 L17 L6 L7 | L4 L5 L28 L0
sketch "Sketch4" plane through (0, 0, 0) normal (0, 0, -1) x (-1, 0, 0)
  line L0 (-330, -92.25) -> (-315, -92.25) projected
  line L1 (-315, -122.25) -> (-330, -122.25) projected
  line L2 (-330, -122.25) -> (-331, -122.25)
  line L3 (-331, -122.25) -> (-331, -116.25)
  line L4 (-331, -116.25) -> (-319.9725, -116.25)
  line L5 (-319.9725, -116.25) -> (-319.9725, -98.25)
  line L6 (-329.7225, -98.25) -> (-317.2225, -98.25) projected
  line L7 (-331, -98.25) -> (-319.9725, -98.25)
  line L8 (-331, -98.25) -> (-331, -92.25)
  line L9 (-331, -92.25) -> (-330, -92.25)
  line L10 (-317.2225, -116.25) -> (-329.7225, -116.25) projected
  line L11 (-313.9725, -92.25) -> (-313.9725, -122.25)
  line L12 (-313.9725, -92.25) -> (-315, -92.25)
  line L13 (-313.9725, -122.25) -> (-315, -122.25)
  line L14 (-316.9725, -114.2775) -> (-316.9725, -100.2725) projected
  point P0 (0, 0)
  dimension "d79" = 3
  dimension "d80" = 3
  constraints: 20 end point, 5 perpendicular, 3 point on line, 2 horizontal, 1 collinear, 1 parallel, 1 vertical
  measures "d79" distance between parallel lines of L11 L14
  measures "d80" distance between parallel lines of L14 L5
extrude "Extrusion4" cut sketch "Sketch4" against normal blind 2
sketch "Sketch5" plane through (274, -126.25, 0) normal (-1, 0, 0) x (0, 0, 1)
  line L0 (0, 19.1) -> (3, 19.1) projected
  line L1 (0, 0) -> (3, 0) projected
  line L2 (3, 19.1) -> (1.5, 19.1)
  line L3 (1.5, 19.1) -> (1.5, 0)
  line L4 (1.5, 0) -> (3, 0)
  line L5 (3, 0) -> (3, 19.1)
  point P0 (0, 126.25)
  constraints: 8 end point, 2 parallel, 1 horizontal, 1 midpoint, 1 perpendicular
extrude "Extrusion5" add sketch "Sketch5" along normal blind 2
sketch "Sketch6" plane through (278.5, -88.05, 0) normal (-1, 0, 0) x (0, 0, 1)
  line L0 (0, 0) -> (3, 0) projected
  line L1 (0.5, 18.55) -> (3, 18.55) projected
  line L2 (3, 0) -> (1.4, 0)
  line L3 (1.4, 0) -> (1.4, 18.55)
  line L4 (1.4, 18.55) -> (3, 18.55)
  line L5 (3, 18.55) -> (3, 0)
  point P0 (0, 88.05)
  point P1 (3, 18.55)
  dimension "d70" = 1.6
  constraints: 8 end point, 2 parallel, 1 horizontal, 1 perpendicular, 1 point on line
  measures "d70" distance of L3.end L4.end
extrude "Extrusion6" cut sketch "Sketch6" against normal blind 2
sketch "Sketch8" plane through (274, -64.25, 0) normal (-1, 0, 0) x (0, 0, 1)
  line L0 (0, 22.25) -> (3, 22.25) projected
  line L1 (0.5, 4.75) -> (3, 4.75) projected
  line L2 (3, 22.25) -> (1.5, 22.25)
  line L3 (1.5, 22.25) -> (1.5, 4.75)
  line L4 (1.5, 4.75) -> (3, 4.75)
  line L5 (3, 4.75) -> (3, 22.25)
  point P0 (0, 64.25)
  dimension "d73" = 1.5
  constraints: 8 end point, 2 parallel, 1 horizontal, 1 perpendicular, 1 point on line
  measures "d73" distance of L4.end L3.end
extrude "Extrusion7" add sketch "Sketch8" along normal blind 2
sketch "Sketch9" plane through (277.25, -163, 0) normal (-1, 0, 0) x (0, 0, 1)
  line L0 (3, 17.65) -> (3, 0) projected
  line L1 (0, 0) -> (3, 0) projected
  line L2 (3, 17.65) -> (1.4, 17.65)
  line L3 (1.4, 17.65) -> (1.4, 0)
  line L4 (1.4, 0) -> (3, 0)
  line L5 (3, 0) -> (3, 17.65)
  point P0 (0, 163)
  dimension "d76" = 1.6
  constraints: 8 end point, 2 parallel, 1 horizontal, 1 perpendicular, 1 point on line
  measures "d76" distance of L4.end L3.end
extrude "Extrusion8" cut sketch "Sketch9" against normal blind 2
sketch "Sketch10" plane through (0, 0, 3) normal (0, 0, 1) x (1, 0, 0)
  line L0 (205.9975, -42) -> (247.7, -42) construction
  line L1 (247.7, -42) -> (247.7, -44.95) construction
  line L2 (252.4, -44.95) -> (247.7, -44.95) construction
  line L3 (252.4, -42) -> (252.4, -44.95) construction
  line L4 (252.4, -42) -> (318.0525, -42) construction
  line L5 (318.0525, -42) -> (318.0525, -44.95) construction
  line L6 (320.5025, -44.95) -> (318.0525, -44.95) construction
  line L7 (320.5025, -39.9) -> (320.5025, -44.95) construction
  line L8 (202.35, -39.9) -> (320.5025, -39.9) construction
  line L9 (202.35, -39.9) -> (202.35, -44.95) construction
  line L10 (205.9975, -44.95) -> (202.35, -44.95) construction
  line L11 (205.9975, -42) -> (205.9975, -44.95) construction
  line L12 (315.2975, -163) -> (253.9975, -163) construction
  line L13 (253.9975, -163) -> (253.9975, -160.05) construction
  line L14 (250.9975, -160.05) -> (253.9975, -160.05) construction
  line L15 (250.9975, -163) -> (250.9975, -160.05) construction
  line L16 (250.9975, -163) -> (234.9975, -163) construction
  line L17 (234.9975, -163) -> (234.9975, -160.05) construction
  line L18 (188.9975, -160.05) -> (234.9975, -160.05) construction
  line L19 (188.9975, -163) -> (188.9975, -160.05) construction
  line L20 (188.9975, -163) -> (163.9975, -163) construction
  line L21 (163.9975, -163) -> (163.9975, -160.05) construction
  line L22 (117.9975, -160.05) -> (163.9975, -160.05) construction
  line L23 (117.9975, -163) -> (117.9975, -160.05) construction
  line L24 (117.9975, -163) -> (77.9475, -163) construction
  line L25 (77.9475, -163) -> (77.9475, -160.05) construction
  line L26 (74.9975, -160.05) -> (77.9475, -160.05) construction
  line L27 (74.9975, -165.1) -> (74.9975, -160.05) construction
  line L28 (318.2475, -165.1) -> (74.9975, -165.1) construction
  line L29 (318.2475, -165.1) -> (318.2475, -160.05) construction
  line L30 (315.2975, -160.05) -> (318.2475, -160.05) construction
  line L31 (315.2975, -163) -> (315.2975, -160.05) construction
  line L32 (320.5025, -59.5) -> (320.5025, -42) projected
  line L33 (317.8525, -42) -> (320.5025, -42)
  line L34 (320.5025, -42) -> (320.5025, -45.15)
  line L35 (320.5025, -45.15) -> (317.8525, -45.15)
  line L36 (317.8525, -45.15) -> (317.8525, -42)
  line L37 (315.0975, -163) -> (318.4475, -163)
  line L38 (318.4475, -163) -> (318.4475, -159.85)
  line L39 (318.4475, -159.85) -> (315.0975, -159.85)
  line L40 (315.0975, -159.85) -> (315.0975, -163)
  point P0 (0, 0)
  dimension "d82" = 0.2
  dimension "d83" = 0.2
  dimension "d84" = 0.2
  dimension "d85" = 0.2
  dimension "d86" = 0.2
  constraints: 16 end point, 4 parallel, 3 point on line, 2 horizontal, 2 perpendicular
  measures "d82" distance between parallel lines of L31 L40
  measures "d83" distance between parallel lines of L39 L30
  measures "d84" distance between parallel lines of L38 L29
  measures "d85" distance between parallel lines of L5 L36
  measures "d86" distance between parallel lines of L35 L6
extrude "Extrusion9" cut sketch "Sketch10" against normal blind 2.5
sketch "Sketch11" plane through (0, 0, 3) normal (0, 0, 1) x (1, 0, 0)
  line L0 (308.9549, -92.9839) -> (312.3112, -92.9839) construction
  line L1 (312.3112, -92.9839) -> (312.3112, -96.0339) construction
  line L2 (312.3112, -96.0339) -> (308.9549, -96.0339) construction
  line L3 (308.9549, -96.0339) -> (308.9549, -92.9839) construction
  line L4 (309.5151, -92.9839) -> (310.2288, -92.9839)
  line L5 (310.2288, -92.9839) -> (310.2288, -97.9839)
  line L6 (310.2288, -97.9839) -> (309.5151, -97.9839)
  line L7 (309.5151, -97.9839) -> (309.5151, -92.9839)
  line L8 (311.3491, -92.9839) -> (312.0628, -92.9839)
  line L9 (312.0628, -92.9839) -> (312.0628, -97.9839)
  line L10 (312.0628, -97.9839) -> (311.3491, -97.9839)
  line L11 (311.3491, -97.9839) -> (311.3491, -92.9839)
  line L12 (313.1831, -92.9839) -> (313.8968, -92.9839)
  line L13 (313.8968, -92.9839) -> (313.8968, -97.9839)
  line L14 (313.8968, -97.9839) -> (313.1831, -97.9839)
  line L15 (313.1831, -97.9839) -> (313.1831, -92.9839)
  point P0 (0, 0)
  constraints: 2 other
extrude "Extrusion10" cut sketch "Sketch11" against normal blind 1
equation "\"d0\" = sw"
equation "\"d1\" = sw"
equation "\"d2\" = sw"
equation "\"d3\" = sw"
equation "\"d4\" = sw"
equation "\"d5\" = sw"
equation "\"d6\" = sw"
equation "\"d7\" = sw"
equation "\"d8\" = sw"
equation "\"d9\" = sw"
equation "\"d10\" = sw"
equation "\"d11\" = sw"
equation "\"d12\" = sw"
equation "\"d13\" = sw"
equation "\"d14\" = sw"
equation "\"d15\" = sw"
equation "\"d16\" = sw"
equation "\"d17\" = sw"
equation "\"d18\" = sw"
equation "\"d19\" = sw"
equation "\"d20\" = sw"
equation "\"d21\" = sw"
equation "\"d22\" = sw"
equation "\"d23\" = sw"
equation "\"d24\" = sw"
equation "\"d25\" = sw"
equation "\"d26\" = sw"
equation "\"d27\" = sw"
equation "\"d28\" = sw"
equation "\"d29\" = sw"
equation "\"d30\" = sw"
equation "\"d31\" = sw"
equation "\"d32\" = sw"
equation "\"d33\" = sw"
equation "\"d34\" = sw"
equation "\"d35\" = sw"
equation "\"d36\" = sw"
equation "\"d37\" = sw"
equation "\"d52\" = d51"
equation "\"d53\" = d51"
equation "\"d83\" = d82"
equation "\"d84\" = d82"
equation "\"d85\" = d82"
equation "\"d86\" = d82"
equation "\"sw\" = 14.005"
body "Solid1"
